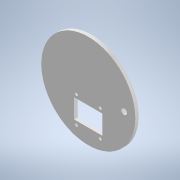
# Autodesk Inventor part: top
Saved by Autodesk Inventor 2022 (Build 260153000, 153)
## iProperties
Created: 2025-06-18
Part Number: top
Material: Типовые
Document SubType Name: Modeling
Designer: korsh624
Density: 1 g/cm^3
Appearance: По умолчанию
Author: korsh624
Autodesk Inventor part; units mm, degrees
ref_plane "YZ Plane" through (0, 0, 0) normal (1, 0, 0) x (0, 1, 0)
ref_plane "XZ Plane" through (0, 0, 0) normal (0, 1, 0) x (-1, 0, 0)
ref_plane "XY Plane" through (0, 0, 0) normal (0, 0, 1) x (1, 0, 0)
sketch "Эскиз3" plane through (0, 0, 0) normal (0, 0, 1) x (1, 0, 0)
  circle A0 centre (0, 0) radius 41.5
  line L0 (12.5, -11.0597) -> (-12.5, -11.0597) projected
  line L1 (-12.5, -11.0597) -> (-12.5, -28.0597) projected
  line L2 (-12.5, -11.0597) -> (12.5, -11.0597)
  line L3 (12.5, -11.0597) -> (12.5, -28.0597)
  line L4 (12.5, -28.0597) -> (-12.5, -28.0597)
  line L5 (-12.5, -28.0597) -> (-12.5, -11.0597)
  dimension "d9" = 83
  dimension "d10" = 25
  dimension "d11" = 17
  dimension "d13" = 25
  dimension "d14" = 17
  dimension "d15" = 12.5
  constraints: 8 end point, 2 parallel, 1 centre point, 1 coincident, 1 horizontal, 1 perpendicular
  measures "d9" diameter of A0
  measures "d10" distance of L0.start L0.end
  measures "d11" distance of L0.end L1.end
  measures "d13" distance of L2.start L2.end
  measures "d14" distance of L2.end L3.end
  measures "d15" distance from line of point (0, 0) L5
extrude "Выдавливание3" add sketch "Эскиз3" along normal blind 3
sketch "Эскиз4" plane through (0, 0, 3) normal (0, 0, 1) x (1, 0, 0)
  arc A0 (5.7629, -8.6636) -> (-4.709, -8.7124) centre (0.4132, 15.7598) ccw
  circle A1 centre (0.4132, 15.7598) radius 1.5338
  point P0 (0, 0)
  constraints: 2 centre point, 2 point on circle, 1 coincident, 4 other
extrude "Выдавливание4" cut sketch "Эскиз4" against normal blind 3
sketch "Эскиз5" plane through (0, 0, 3) normal (0, 0, 1) x (1, 0, 0)
  line L0 (-51.8221, -46.0116) -> (-45.155, -49.3714) projected
  circle A0 centre (31.5626, 0.0623) radius 2.5
  point P0 (0, 0)
  dimension "d20" = 5
  constraints: 1 centre point
  measures "d20" diameter of A0
extrude "Выдавливание5" cut sketch "Эскиз5" against normal blind 3
sketch "Эскиз6" plane through (0, 0, 3) normal (0, 0, 1) x (1, 0, 0)
  circle A0 centre (0.4132, 15.7598) radius 1.5338 projected
  point P0 (0, 0)
extrude "Выдавливание6" add sketch "Эскиз6" against normal blind 3
sketch "Эскиз7" plane through (0, 0, 3) normal (0, 0, 1) x (1, 0, 0)
  circle A0 centre (10.5, -7.8097) radius 1.25 projected
  circle A1 centre (-10.5, -7.8097) radius 1.25 projected
  circle A2 centre (-10.5, -31.3097) radius 1.25 projected
  circle A3 centre (10.5, -31.3097) radius 1.25 projected
  point P0 (0, 0)
extrude "Выдавливание7" cut sketch "Эскиз7" against normal blind 3
sketch "Эскиз13" plane through (0, 0, 3) normal (0, 0, 1) x (1, 0, 0)
  circle A0 centre (0, 0) radius 41.5 projected
  circle A1 centre (0, 0) radius 41.7806
  point P0 (-26.934, 31.9403)
  constraints: 1 coincident, 4 other
extrude "Выдавливание12" add sketch "Эскиз13" against normal blind 3
sketch "Эскиз14" plane through (0, 0, 0) normal (0, 0, -1) x (-1, 0, 0)
  circle A0 centre (-24.602, 9.2303) radius 1.6 projected
  circle A1 centre (12.434, 2.9402) radius 1.6 projected
  point P0 (0, 0)
extrude "Выдавливание13" cut sketch "Эскиз14" against normal blind 3
equation "\"d13\" = d10"
equation "\"d14\" = d11"
equation "\"d15\" = 0.5 * d13"
